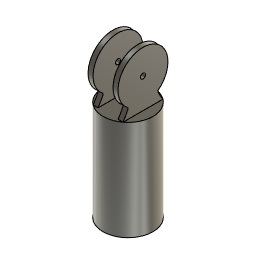
robotarm (Autodesk Fusion 360 archive; units mm, degrees)
design "arm"
Autodesk Fusion 360 part; units mm, degrees
cylinder "CylinderPrimitive1" add diameter 100 height 200 placed x (1, 0, 0) y (0, 1, 0) z (0, 0, 1) at (0, 0, 0) makes body 1
cylinder "CylinderPrimitive1'" add diameter 100 height 50 placed x (1, 0, 0) y (0, 1, 0) z (0, 0, 1) at (0, 0, 0) separate body makes body 2 in component "joint v1"
sketch "Sketch2" plane through (0, 0, 50) normal (0, 0, 1) x (-1, 0, 0) in component "joint v1"
  circle A0 centre (0, 0) radius 50
  line L0 (30, -55) -> (20, -55)
  line L1 (20, -55) -> (20, 55)
  line L2 (20, 55) -> (30, 55)
  line L3 (30, 55) -> (30, -55)
  line L4 (-20, -55) -> (-30, -55)
  line L5 (-30, -55) -> (-30, 55)
  line L6 (-30, 55) -> (-20, 55)
  line L7 (-20, 55) -> (-20, -55)
  constraint horizontal L0
  constraint vertical L1
  constraint horizontal L2
  constraint vertical L3
  constraint horizontal L4
  constraint vertical L5
  constraint horizontal L6
  constraint vertical L7
extrude "Extrude1" add sketch "Sketch2" along normal blind 20 contours A0 L1 L3 | A0 L5 L7 bodies 2 in component "joint v1"
sketch "Sketch3" plane through (0, 0, 0) normal (1, 0, 0) x (0, 1, 0) in component "joint v1"
sketch "Sketch4" plane through (0, 0, 0) normal (0, 1, 0) x (1, 0, 0) in component "joint v1"
sketch "Sketch5" plane through (0, 0, 0) normal (1, 0, 0) x (0, 1, 0) in component "joint v1"
sketch "Sketch6" plane through (-30, 0, 0) normal (-1, 0, 0) x (0, -1, 0) in component "joint v1"
  line L0 (-40, 50) -> (40, 50)
  line L1 (40, 50) -> (40, 70)
  line L2 (40, 70) -> (-40, 70)
  line L3 (-40, 70) -> (-40, 50)
  circle A0 centre (0, 110) radius 50
extrude "Extrude2" cut sketch "Sketch6" against normal blind 100 contours L2 A0 picked at (-7.9978, 68.711) bodies 2 in component "joint v1"
extrude "Extrude3" add sketch "Sketch6" against normal blind 10 contours L2 A0 | L2 A0 bodies 2 in component "joint v1"
sketch "Sketch7" plane through (-30, 0, 0) normal (-1, 0, 0) x (0, -1, 0) in component "joint v1"
  spline S0 degree 5 poles (-35, 70) (-34.486, 70.22) (-33.5207, 70.5968) (-32.2607, 70.9721) (-30.9632, 71.0862) (-30.0086, 70.5551) (-29.7454, 69.3258) (-30.1498, 67.4223) (-31.1578, 64.9093) (-32.6968, 61.8602) (-34.6989, 58.3433) (-36.6299, 55.1973) (-38.2494, 52.6648) (-39.404, 50.9009) (-40, 50) knots 0 0 0 0 0 0 0.1 0.2 0.3 0.4 0.5 0.6 0.7 0.8 0.9 1 1 1 1 1 1
  line L0 (-30, 70) -> (-40, 70)
  line L1 (-40, 70) -> (-46, 70)
  line L2 (-46, 70) -> (-46, 50)
  line L3 (-46, 50) -> (-40, 50)
  point P0 (-30, 70)
  constraint coincident P0 L0.start
  constraint horizontal L0
  constraint perpendicular L1 L2
extrude "Extrude4" cut sketch "Sketch7" against normal blind 100 contours S0 L0 L1 L2 L3 bodies 2 in component "joint v1"
hole "Hole1" at (-30, 0, 110) direction (1, 0, 0) diameter 10 depth 25 tip angle 118 bodies 2 in component "joint v1"
extrude "Extrude5" add sketch "Sketch6" along normal blind 10 separate body contours L2 A0 | L2 A0 makes body 3 in component "joint v1"
move_body "Move1" bodies 3 to x (1, 0, 0) y (0, 1, 0) z (0, 0, 1) at (60, 0, 0) in component "joint v1"
combine "Combine1" operation add target body 3 tool bodies 2 in component "joint v1"
hole "Hole2" at (30, 0, 110) direction (-1, 0, 0) diameter 10 depth 25 tip angle 180 bodies 3 in component "joint v1"
sketch "Sketch8" plane through (0, 0, 0) normal (1, 0, 0) x (0, 1, 0) in component "joint v1"
  line L0 (-35, 70) -> (-50, 70)
  line L1 (-50, 70) -> (-50, 50)
  line L2 (-50, 50) -> (-40, 50)
  spline S0 degree 5 poles (-30, 70) (-29.9562, 69.858) (-29.8764, 69.4532) (-29.8915, 68.6537) (-30.2258, 67.2328) (-31.1578, 64.9093) (-32.6968, 61.8602) (-34.6989, 58.3433) (-36.6299, 55.1973) (-38.2494, 52.6648) (-39.404, 50.9009) (-40, 50) knots 0.337709 0.337709 0.337709 0.337709 0.337709 0.337709 0.4 0.5 0.6 0.7 0.8 0.9 1 1 1 1 1 1
  line L3 (-30.2187, 70.7091) -> (-29.7813, 69.2909)
  line L4 (-30, 70) -> (-50, 70)
  line L5 (-50, 50) -> (-40, 50)
  constraint horizontal L0
  constraint perpendicular L0 L1
  constraint perpendicular L1 L2
  constraint midpoint S0.start L3
  constraint perpendicular L1 L4
extrude "Extrude6" cut sketch "Sketch8" along normal blind 45 and the other way blind 54 bodies 3 in component "joint v1"
combine "Combine1'" operation add target body 1 tool bodies 3 body 3 seen with x (1, 0, 0) y (0, 1, 0) z (0, 0, 1) at (0, 0, 150) keep tools
combine "Combine2" operation add target body 1 tool bodies 3 body 3 seen with x (1, 0, 0) y (0, 1, 0) z (0, 0, 1) at (0, 0, 150) keep tools
move_body "Move1'" bodies 1 to x (1, 0, 0) y (0, 1, 0) z (0, 0, 1) at (275, 0, 0)
move_body "Move2" bodies 1 to x (1, 0, 0) y (0, 1, 0) z (0, 0, 1) at (-275, 0, 0)

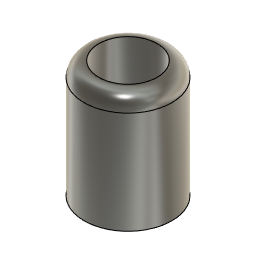
design "base_link"
Autodesk Fusion 360 part; units mm, degrees
cylinder "CylinderPrimitive1" add diameter 150 height 100 placed x (1, 0, 0) y (0, 1, 0) z (0, 0, 1) at (0, 0, 0)
fillet "Fillet1" radius 25 1 faces at (18.6055, 20.7304, 100)
extrude "Extrude2" add 1 faces at (18.6055, 20.7304, 0) along direction (0, 0, -1) blind 100
extrude "Extrude3" cut 1 faces at (-13.5518, -2.484, 100) along direction (0, 0, 1) blind -380 and the other way blind -130
move_body "Move1" bodies 1 to x (1, 0, 0) y (0, 1, 0) z (0, 0, 1) at (0, 0, 100)
move_body "Move2" bodies 1 to x (1, 0, 0) y (0, 1, 0) z (0, 0, 1) at (0, 0, -100)
move_body "Move3" bodies 1 to x (1, 0, 0) y (0, 1, 0) z (0, 0, 1) at (0, 0, 100)
